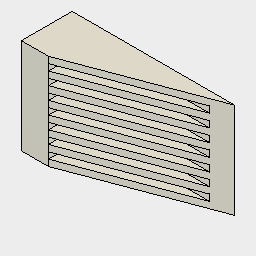
hodor v1 (Autodesk Fusion 360 design; units mm, degrees)
Autodesk Fusion 360 part; units mm, degrees
sketch "Sketch1" plane through (0, 0, 0) normal (0, 1, 0) x (1, 0, 0)
  line L0 (-24, 0) -> (24, 0)
  line L1 (1.75, 0) -> (22.5, 0)
  line L2 (0, -1.75) -> (0, -22.5)
  line L3 (-24, 0) -> (-24, -15)
  line L4 (-24, -15) -> (-16, -15)
  line L5 (-16, -15) -> (24, 0)
  dimension "d1" = 48
  dimension "d2" = 15
  dimension "d3" = 8
  measures "d1" distance of L0.start L0.end
  measures "d2" distance of L0.start L3.end
  measures "d3" distance of L3.end L4.end
extrude "Extrude1" add sketch "Sketch1" along normal blind 28.2
ref_plane "WorkPlane1" through (0, 1.88, 7.5) normal (0, -1, 0) x (-1, 0, 0)
sketch "Sketch2" plane through (0, 1.88, 7.5) normal (0, -1, 0) x (1, 0, 0)
  line L0 (-16, 7.5) -> (24, -7.5)
  line L1 (24, -7.5) -> (-24, -7.5)
  line L2 (18.6667, -5.5) -> (-16, -5.5)
  line L3 (-16, -5.5) -> (-16, 7.5)
  line L4 (18.6667, 7.5) -> (-16, 7.5)
  line L5 (18.6667, -5.5) -> (18.6667, 7.5)
  dimension "d7" = 2
  measures "d7" distance of L1 L2.start
extrude "Extrude2" cut sketch "Sketch2" against normal blind 1.88
pattern_linear "R-Pattern1" count 7 spacing 3.76 along (0, 1, 0) of "Extrude2"
equation "d4 = ( ( 1.88 * 2 ) * 1 mm ) * 7 + 1.88 mm"
equation "d12 = -1.88 * 2 mm"
